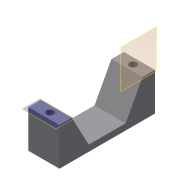
# Autodesk Inventor part: 30_CUBE_openSIM_Lensfixation
Saved by Autodesk Inventor 2019 (Build 230136000, 136)
## iProperties
Created: 2020-03-03
Part Number: 30_CUBE_openSIM_Lensfixation
Material: Generic
Document SubType Name: Modeling
Designer: diederichbenedict
Density: 1 g/cm^3
Appearance: Default
Author: diederichbenedict
Autodesk Inventor part; units mm, degrees
ref_plane "YZ Plane" through (0, 0, 0) normal (1, 0, 0) x (0, 1, 0)
ref_plane "XZ Plane" through (0, 0, 0) normal (0, 1, 0) x (-1, 0, 0)
ref_plane "Work Plane1" through (182.8, -16.921, -7.958) normal (0, -1, 0) x (0, 0, -1)
ref_plane "Work Plane2" through (182.8, -6.9868, -42.1222) normal (1, 0, 0) x (0, 0, -1)
sketch "Sketch1" plane through (182.8, -6.9868, -42.1222) normal (1, 0, 0) x (0, 0, -1)
  arc A0 (5.0194, 6.9868) -> (5.8778, 5.8182) centre (7.8778, 8.1868) ccw projected
  line L0 (-9.7772, 6.9868) -> (5.0194, 6.9868) projected
  arc A1 (-7.9865, 5.8774) -> (-9.7772, 6.9868) centre (-9.7772, 4.9868) ccw projected
  line L1 (-7.9865, 5.8774) -> (-0.1222, -9.9342) projected
  line L2 (-0.1222, -9.9342) -> (5.8778, -9.9342) projected
  line L3 (5.8778, -9.9342) -> (5.8778, 5.8182) projected
  line L4 (-42.1222, 6.9868) -> (-42.1222, -9.9342) projected
  line L5 (-42.1222, -9.9342) -> (-34.1642, -9.9342) projected
  line L6 (-34.1642, -9.9342) -> (-26.2998, 5.8774) projected
  arc A2 (-24.5091, 6.9868) -> (-26.2998, 5.8774) centre (-24.5091, 4.9868) ccw projected
  line L7 (-42.1222, 6.9868) -> (-24.5091, 6.9868) projected
  circle A3 centre (-17.1432, -9.9342) radius 15.24 construction
  line L8 (-17.1432, -9.9342) -> (-17.1432, -20.9232) construction
  line L9 (-17.1432, -9.9342) -> (-6.1542, -9.9342) construction
  line L10 (-0.1222, -9.9342) -> (-8.2255, -25.1742)
  line L11 (-0.1222, -9.9342) -> (17.1381, -9.9342) construction
  line L12 (-8.2255, -25.1742) -> (-17.1432, -25.1742)
  line L13 (-17.1432, -25.1742) -> (-17.1432, -28.1742)
  line L14 (-17.1432, -28.1742) -> (5.8778, -28.1742)
  line L15 (5.8778, -28.1742) -> (5.8778, -9.9342)
  line L16 (-0.1222, -9.9342) -> (5.8778, -9.9342)
  dimension "d0" = 90
  dimension "d1" = 118
  dimension "d2" = 3
  dimension "d3" = 90
  constraints: 18 end point, 3 horizontal, 2 equal length, 1 collinear, 1 perpendicular, 1 vertical, 1 vertical alignment, 1 other
  measures "d0" angle of L8 L9
  measures "d1" angle of L10 L11
  measures "d2" distance of L12.end L13.end
  measures "d3" angle of L14 L13
ref_plane "Work Plane3" through (167.8, -16.921, -48) normal (-1, 0, 0) x (0, 0, 1)
extrude "Extrusion1" add sketch "Sketch1" against normal up to surface (15 mm away) contours L15 L14 L13 L12 L10 L2
sketch "Sketch2" plane through (182.8, -35.161, -48) normal (0, -1, 0) x (1, 0, 0)
  circle A0 centre (-7.5, 3) radius 1.45 projected
  point P0 (-182.8, 48)
hole "Hole1" at (175.3, -35.161, -45) direction (0, 1, 0) diameter 3.5 end through all counterbore diameter 6 counterbore depth 6.5
mirror "Mirror1" about plane through (182.8, -35.161, -24.979) normal (0, 0, 1) of "Extrusion1", "Hole1"
body "Solid1"
